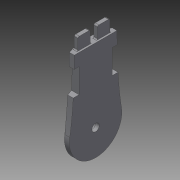
# Autodesk Inventor part: mid_curveLpin
Saved by Autodesk Inventor 2014 (Build 180170000, 170)
## iProperties
Created: 2014-04-24
Part Number: mid_curveLpin
Material: Generic
Document SubType Name: Modeling
Designer: t_emanb
Density: 1 g/cm^3
Appearance: Default
Author: t_emanb
Autodesk Inventor part; units mm, degrees
ref_plane "YZ Plane" through (0, 0, 0) normal (1, 0, 0) x (0, 1, 0)
ref_plane "XZ Plane" through (0, 0, 0) normal (0, 1, 0) x (-1, 0, 0)
sketch "Sketch1" plane through (0, 0, 0) normal (1, 0, 0) x (0, 1, 0)
  line L0 (0, -22.225) -> (152.4, -22.225) construction
  line L1 (152.4, -22.225) -> (152.4, 22.225) construction
  line L2 (152.4, 22.225) -> (0, 22.225) construction
  line L3 (0, 22.225) -> (0, -22.225) construction
  line L4 (0, 0) -> (152.4, 0) construction
  arc A0 (0, 22.225) -> (0, -22.225) centre (0, 0) ccw construction
  arc A1 (152.4, -22.225) -> (152.4, 22.225) centre (152.4, 0) ccw construction
  circle A2 centre (0, 0) radius 2.95 construction
  circle A3 centre (152.4, 0) radius 2.95 construction
  arc A4 (4.446041, 26.940597) -> (4.446041, -26.940597) centre (0, 0) ccw
  line L5 (76.2, 22.225) -> (76.2, -22.225)
  line L6 (4.446041, 26.940597) -> (33.02, 22.225) construction
  line L7 (33.02, 22.225) -> (76.2, 22.225) construction
  spline S0 degree 2 poles (4.446041, 26.940597) (33.02, 22.225) (76.2, 22.225) knots 1 1 1 2 2 2
  line L8 (33.02, 22.225) -> (33.02, 0) construction
  line L9 (4.446041, -26.940597) -> (33.02, -22.225) construction
  line L10 (33.02, -22.225) -> (76.2, -22.225) construction
  spline S1 degree 2 poles (4.446041, -26.940597) (33.02, -22.225) (76.2, -22.225) knots 1 1 1 2 2 2
  dimension "d0" = 152.4
  dimension "d1" = 44.45
  dimension "d2" = 5.9
  dimension "d4" = 5.08
  dimension "d9" = 43.18
  constraints: 14 end point, 7 coincident, 6 point on circle, 5 centre point, 4 midpoint, 2 horizontal, 2 parallel, 2 perpendicular, 2 symmetric about line, 1 equal radius, 1 point on line, 7 other
  measures "d0" distance of L2.end L1.end
  measures "d1" distance of L2.end L0.start
  measures "d2" diameter of A2
  measures "d4" radial gap between concentric circles of A0 A4
  measures "d9" distance between parallel lines of L8 L5
extrude "Extrusion1" add sketch "Sketch1" along normal blind 5.08
sketch "Sketch2" plane through (0, 0, 0) normal (-1, 0, 0) x (0, 0, 1)
  arc A0 (-26.940597, 4.446041) -> (26.940597, 4.446041) centre (0, 0) ccw
  circle A1 centre (0, 0) radius 27.305
  line L0 (27.305, 0) -> (-27.305, 0)
  constraints: 4 point on circle, 2 end point, 1 centre point, 1 coincident, 1 concentric, 1 horizontal, 1 midpoint
ref_plane "Work Plane1" through (0, 0, 27.305) normal (0, 1, 0) x (0, 0, -1)
sketch "Sketch3" plane through (0, 0, 27.305) normal (0, 1, 0) x (0, 0, -1)
  line L0 (54.245597, 0) -> (0.364403, 0)
  line L1 (54.245597, 0) -> (54.245597, -5.08)
  line L2 (0.364403, -5.08) -> (54.245597, -5.08)
  line L3 (0.364403, 0) -> (0.364403, -5.08)
  line L4 (27.305, -5.08) -> (27.305, 6.35) construction
  line L5 (0.364403, 0) -> (54.245597, 0)
  line L6 (54.61, 0) -> (54.61, -5.08)
  line L7 (0, 0) -> (0, -5.08)
  arc A0 (54.61, 0) -> (0, 0) centre (27.305, -55.53075) ccw
  line L8 (0, 0) -> (54.61, 0)
  point P0 (27.305, 0)
  dimension "d13" = 11.43
  constraints: 6 end point, 3 point on circle, 1 centre point, 1 collinear, 1 midpoint, 1 perpendicular
  measures "d13" distance of L4.start L4.end
sketch "Sketch4" plane through (0, 76.2, 22.225) normal (0, 1, 0) x (1, 0, 0)
  line L0 (5.08, 44.45) -> (5.08, 0)
  arc A0 (0, 44.45) -> (0, 0) centre (62.917917, 22.225) ccw
  line L1 (5.08, 22.225) -> (-3.81, 22.225) construction
  line L2 (0, 0) -> (0, 44.45)
  point P0 (0, 22.225)
  dimension "d14" = 8.89
  constraints: 4 end point, 3 point on circle, 1 centre point, 1 midpoint
  measures "d14" distance of L1.start L1.end
loft "Loft1" add profiles "Sketch3", "Sketch4" contours L0 L8 A0 / all
extrude "Extrusion2" cut sketch "Sketch2" along normal through all contours A1 A0 L0
sketch "Sketch5" plane through (5.08, 0, 0) normal (1, 0, 0) x (0, 0, -1)
  line L0 (22.225, 76.2) -> (-22.225, 76.2)
  spline S0 degree 2 poles (-22.225, 76.2) (-22.225, 33.02) (-26.940597, 4.446041) knots 0 0 0 1 1 1
  arc A0 (-26.940597, 4.446041) -> (26.940597, 4.446041) centre (0, 0) ccw
  spline S1 degree 2 poles (26.940597, 4.446041) (22.225, 33.02) (22.225, 76.2) knots 0 0 0 1 1 1
  line L1 (-27.304944, -0.055527) -> (-27.304944, 76.2)
  line L2 (-27.304944, 76.2) -> (-22.225, 76.2)
  line L3 (22.225, 76.2) -> (27.305, 76.2)
  line L4 (27.305, 76.2) -> (27.305, 0)
  constraints: 8 end point, 2 perpendicular, 2 point on circle, 1 collinear, 1 tangent, 1 vertical, 2 other
sketch "Sketch5 outline for Extrusion3" plane through (5.08, 0, 0) normal (1, 0, 0) x (0, 0, -1)
  spline S0 degree 2 poles (26.940597, 4.446041) (22.225, 33.02) (22.225, 76.2) knots 0 0 0 1 1 1
  line L0 (27.305, 76.2) -> (22.225, 76.2)
  line L1 (27.305, 0) -> (27.305, 76.2)
  arc A0 (26.940597, 4.446041) -> (27.305, 0) centre (0, 0) cw
  spline S1 degree 2 poles (-22.225, 76.2) (-22.225, 33.02) (-26.940597, 4.446041) knots 0 0 0 1 1 1
  arc A1 (-26.940597, 4.446041) -> (-27.304944, -0.055527) centre (0, 0) ccw
  line L2 (-27.304944, 76.2) -> (-27.304944, -0.055527)
  line L3 (-22.225, 76.2) -> (-27.304944, 76.2)
extrude "Extrusion3" cut sketch "Sketch5 outline for Extrusion3" against normal through all
sketch "Sketch6" plane through (5.08, 76.2, 22.225) normal (0, 1, 0) x (1, 0, 0)
  line L0 (0, 44.45) -> (0, 0)
  arc A0 (-5.08, 44.45) -> (-5.08, 0) centre (57.837917, 22.225) ccw
  line L1 (-5.588, 38.7985) -> (-1.778, 38.7985)
  line L2 (-1.778, 38.7985) -> (-1.778, 25.9715)
  line L3 (-1.778, 25.9715) -> (-5.588, 25.9715)
  line L4 (-5.588, 25.9715) -> (-5.588, 38.7985)
  line L5 (-8.89, 22.225) -> (0, 22.225) construction
  line L6 (-5.588, 5.6515) -> (-1.778, 5.6515)
  line L7 (-1.778, 5.6515) -> (-1.778, 18.4785)
  line L8 (-1.778, 18.4785) -> (-5.588, 18.4785)
  line L9 (-5.588, 18.4785) -> (-5.588, 5.6515)
  point P0 (-5.08, 22.225)
  dimension "d24" = 3.81
  dimension "d25" = 1.778
  dimension "d44" = 12.827
  dimension "d45" = 7.493
  constraints: 18 end point, 4 symmetric about line, 2 parallel, 1 horizontal, 1 midpoint, 1 perpendicular, 1 point on circle
  measures "d24" distance of L1.start L1.end
  measures "d25" distance between parallel lines of L0 L2
  measures "d44" distance of L1.end L2.end
  measures "d45" distance between parallel lines of L3 L8
extrude "Extrusion4" add sketch "Sketch6" along normal blind 12.7
sketch "Sketch7" plane through (5.08, 0, 0) normal (1, 0, 0) x (0, 0, -1)
  line L0 (22.225, 76.2) -> (-22.225, 76.2)
  spline S0 degree 2 poles (-22.225, 76.2) (-22.225, 33.02) (-26.940597, 4.446041) knots 0 0 0 1 1 1
  arc A0 (-26.940597, 4.446041) -> (26.940597, 4.446041) centre (0, 0) ccw
  spline S1 degree 2 poles (26.940597, 4.446041) (22.225, 33.02) (22.225, 76.2) knots 0 0 0 1 1 1
  line L1 (-22.334611, 63.373) -> (-17.254611, 63.373)
  line L2 (-17.254611, 63.373) -> (-17.254611, 38.1)
  line L3 (-17.254611, 38.1) -> (-23.312252, 38.1)
  line L4 (23.312252, 38.1) -> (17.254611, 38.1)
  line L5 (17.254611, 38.1) -> (17.254611, 63.373)
  line L6 (17.254611, 63.373) -> (22.334611, 63.373)
  dimension "d28" = 5.08
  dimension "d29" = 5.08
  dimension "d30" = 38.1
  dimension "d31" = 25.273
  constraints: 12 end point, 3 collinear, 3 parallel, 2 perpendicular, 6 other
  measures "d28" distance of L1.start L1.end
  measures "d29" distance of L5.end L6.end
  measures "d30" distance from line of A0.centre L3
  measures "d31" distance of L1.end L2.end
extrude "Extrusion5" cut sketch "Sketch7" against normal through all contours S1 L4 L5 L6 | L1 L2 L3 S0
sketch "Sketch9" plane through (0, 0, 0) normal (-1, 0, 0) x (0, 0, 1)
  arc A0 (-26.940597, 4.446041) -> (26.940597, 4.446041) centre (0, 0) ccw
  circle A1 centre (0, 0) radius 20.32
  arc A2 (-26.940597, 4.446041) -> (26.940597, 4.446041) centre (0, 0) ccw
  arc A3 (26.940597, 4.446041) -> (-26.940597, 4.446041) centre (0, 0) ccw
  dimension "d37" = 40.64
  constraints: 2 centre point, 2 point on circle, 1 coincident
  measures "d37" diameter of A1
extrude "Extrusion7" add sketch "Sketch9" along normal blind 5.08 contours A1
fillet "Fillet1" radius 3.175 2 edges at (-5.08, 0, -20.32) (0, 0, -20.32)
sketch "Sketch10" plane through (0, 0, 0) normal (0, 0, 1) x (1, 0, 0)
  line L0 (5.08, 76.2) -> (5.08, 4.446041)
  line L1 (5.08, -27.305) -> (5.08, 4.446041)
  line L2 (-5.08, -17.145) -> (-5.08, 17.145)
  line L3 (5.08, 0) -> (-5.08, 0)
  line L4 (5.08, -3.8735) -> (1.2065, -3.8735)
  arc A0 (-2.667, 0) -> (1.2065, -3.8735) centre (1.2065, 0) ccw
  point P0 (0, 0)
  point P1 (5.08, 38.1)
  dimension "d41" = 7.747
  dimension "d42" = 3.8735
  constraints: 4 end point, 4 point on line, 2 midpoint, 2 point on circle, 1 centre point, 1 parallel, 1 tangent
  measures "d41" distance of L3.start A0.start
  measures "d42" distance between parallel lines of L3 L4
revolve "Revolution1" cut sketch "Sketch10" angle 360 about axis through (5.08, 0, 0) along (-1, 0, 0)
fillet "Fillet2" radius 1.397 4 edges at (1.397, 88.9, 16.5735) (1.397, 88.9, 3.7465) (1.397, 88.9, -3.7465) (1.397, 88.9, -16.5735)
fillet "Fillet3" radius 1.143 4 edges at (1.397, 76.2, 16.5735) (1.397, 76.2, 3.7465) (1.397, 76.2, -3.7465) (1.397, 76.2, -16.5735)
body "Solid1"
